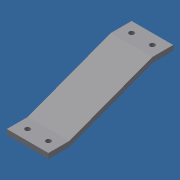
# Autodesk Inventor part: BracketControlPannel
Saved by Autodesk Inventor 2021 (Build 250183000, 183)
## iProperties
Created: 2022-09-10
Part Number: BracketControlPannel
Material: Generic
Document SubType Name: Modeling
Designer: Nathann
Density: 1 g/cm^3
Appearance: Default
Author: Nathann
Autodesk Inventor part; units mm, degrees
ref_plane "YZ Plane" through (0, 0, 0) normal (1, 0, 0) x (0, 1, 0)
ref_plane "XZ Plane" through (0, 0, 0) normal (0, 1, 0) x (-1, 0, 0)
ref_plane "XY Plane" through (0, 0, 0) normal (0, 0, 1) x (1, 0, 0)
sketch "Sketch1" plane through (0, 0, 0) normal (1, 0, 0) x (0, 1, 0)
  line L0 (0, 0) -> (5, 0)
  line L1 (5, 0) -> (5, 20)
  line L2 (5, 20) -> (0, 20)
  line L3 (0, 20) -> (0, 0)
  line L4 (-25, 100) -> (-30, 100)
  line L5 (-30, 100) -> (-30, 120)
  line L6 (-30, 120) -> (-25, 120)
  line L7 (-25, 120) -> (-25, 100)
  line L8 (5, 20) -> (-25, 100)
  line L9 (0, 20) -> (-30, 100)
  dimension "d0" = 5
  dimension "d1" = 20
  dimension "d2" = 5
  dimension "d3" = 20
  dimension "d4" = 35
  dimension "d5" = 120
  constraints: 20 end point, 4 parallel, 2 horizontal, 2 perpendicular
  measures "d0" distance of L0.start L0.end
  measures "d1" distance of L2.end L0.start
  measures "d2" distance of L5.end L6.end
  measures "d3" distance of L4.end L5.end
  measures "d4" distance between parallel lines of L5 L1
  measures "d5" distance between parallel lines of L6 L0
extrude "Extrusion1" add sketch "Sketch1" along normal blind 40
sketch "Sketch2" plane through (0, 0, 0) normal (0, -1, 0) x (1, 0, 0)
  circle A0 centre (30, 10) radius 2.5
  circle A1 centre (10, 10) radius 2.5
  circle A2 centre (30, 110) radius 2.5
  circle A3 centre (10, 110) radius 2.5
  line L0 (40, 120) -> (40, 100) projected
  line L1 (0, 120) -> (40, 120) projected
  line L2 (0, 120) -> (0, 100) projected
  line L3 (0, 20) -> (0, 0) projected
  line L4 (40, 20) -> (40, 0) projected
  line L5 (0, 0) -> (40, 0) projected
  dimension "d8" = 5
  dimension "d9" = 5
  dimension "d10" = 5
  dimension "d11" = 5
  dimension "d12" = 10
  dimension "d13" = 10
  dimension "d14" = 10
  dimension "d15" = 10
  dimension "d16" = 10
  dimension "d17" = 10
  dimension "d18" = 10
  dimension "d19" = 10
  constraints: 4 centre point
  measures "d8" diameter of A0
  measures "d9" diameter of A1
  measures "d10" diameter of A3
  measures "d11" diameter of A2
  measures "d12" distance from line of L0 A2.centre
  measures "d13" distance from line of L1 A2.centre
  measures "d14" distance from line of L1 A3.centre
  measures "d15" distance from line of L2 A3.centre
  measures "d16" distance from line of L3 A1.centre
  measures "d17" distance from line of L4 A0.centre
  measures "d18" distance from line of L5 A0.centre
  measures "d19" distance from line of A1.centre L5
extrude "Extrusion2" cut sketch "Sketch2" against normal mid plane 90
body "Solid1"
